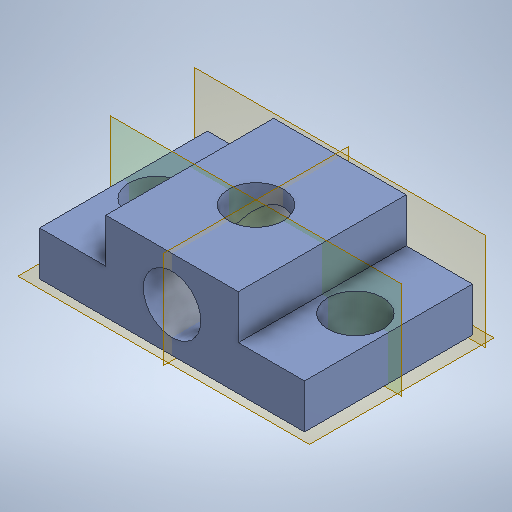
# Autodesk Inventor part: suporte_veio_001_001
Saved by Autodesk Inventor 2026 (Build 300175000, 175)
## iProperties
Created: 2025-04-09
Part Number: suporte_veio_001_001
Material: Aluminum 6061
Document SubType Name: Modeling
Designer: Carlos Dias
Density: 2.7 g/cm^3
Appearance: Rubber - Blue
Author: Carlos Dias
Autodesk Inventor part; units mm, degrees
sketch "Sketch1" plane through (0, 0, 0) normal (0, 0, 1) x (1, 0, 0)
  line L0 (-15, 0) -> (15, 0)
  line L1 (-15, 5) -> (-15, 0)
  line L2 (15, 5) -> (15, 0)
  line L3 (15, 5) -> (7.5, 5)
  line L4 (-15, 5) -> (-7.5, 5)
  line L5 (-7.5, 5) -> (-7.5, 10)
  line L6 (7.5, 5) -> (7.5, 10)
  line L7 (7.5, 10) -> (-7.5, 10)
  point P0 (0, 0)
  point P1 (0, 0)
  dimension "d0" = 30
  dimension "d1" = 5
  dimension "d2" = 15
  constraints: 16 end point, 4 equal length, 4 horizontal, 4 vertical, 2 coincident, 1 midpoint
  measures "d0" distance of L0.start L0.end
  measures "d1" distance of L1.start L0.start
  measures "d2" distance between parallel lines of L6 L5
extrude "Extrusion1" add sketch "Sketch1" along normal blind 19
sketch "Sketch2" plane through (-15, 5, 0) normal (0, 1, 0) x (1, 0, 0)
  circle A0 centre (3.75, -9.5) radius 3.1
  line L0 (0, 0) -> (30, 0) projected
  line L1 (0, 0) -> (0, -19) projected
  line L2 (0, 0) -> (0, -19)
  line L3 (0, 0) -> (7.5, 0)
  point P0 (15, 0)
  point P1 (0, -9.5)
  point P2 (3.75, 0)
  dimension "d5" = 6.2
  constraints: 4 end point, 2 midpoint, 1 centre point, 1 coincident, 1 collinear, 1 horizontal, 1 horizontal alignment, 1 vertical alignment
  measures "d5" diameter of A0
extrude "Extrusion2" cut sketch "Sketch2" against normal through all
mirror "Mirror1" about plane through (0, 0, 0) normal (1, 0, 0) of "Extrusion2"
sketch "Sketch3" plane through (0, 0, 19) normal (0, 0, 1) x (1, 0, 0)
  circle A0 centre (0, 5) radius 3.25
  line L0 (-15, 0) -> (15, 0) projected
  point P0 (0, 0)
  point P1 (0, 0)
  point P2 (-7.5, 5)
  dimension "d9" = 6.5
  constraints: 1 centre point, 1 horizontal alignment, 1 midpoint, 1 vertical alignment
  measures "d9" diameter of A0
extrude "Extrusion3" cut sketch "Sketch3" against normal through all
sketch "Sketch4" plane through (-7.5, 10, 0) normal (0, 1, 0) x (1, 0, 0)
  circle A0 centre (7.5, -9.5) radius 3.1
  line L0 (15, 0) -> (0, 0) projected
  line L1 (0, 0) -> (0, -19) projected
  point P0 (7.5, 0)
  point P1 (7.5, 0)
  point P2 (0, -9.5)
  dimension "d12" = 6.2
  constraints: 2 midpoint, 1 centre point, 1 horizontal alignment, 1 vertical alignment
  measures "d12" diameter of A0
extrude "Extrusion4" cut sketch "Sketch4" against normal up to next
ref_plane "Work Plane1" through (0, 0, 9.5) normal (0, 0, -1) x (-1, 0, 0)
body "Solid1"
